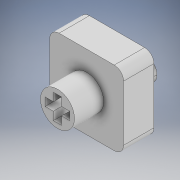
# Autodesk Inventor part: IPC CRUS 5 key
Saved by Autodesk Inventor 2022 (Build 260153000, 153)
## iProperties
Created: 2021-12-31
Part Number: IPC CRUS 5 key
Material: Generic
Document SubType Name: Modeling
Designer: solor
Density: 1 g/cm^3
Appearance: Default
Author: solor
Autodesk Inventor part; units mm, degrees
ref_plane "YZ Plane" through (0, 0, 0) normal (1, 0, 0) x (0, 1, 0)
ref_plane "XZ Plane" through (0, 0, 0) normal (0, 1, 0) x (-1, 0, 0)
sketch "Sketch1" plane through (0, 0, 0) normal (0, 0, 1) x (1, 0, 0)
  line L0 (14.6962, 12.74) -> (14.6962, 0) construction
  line L1 (10.61, 12.2) -> (1.53, 12.2)
  arc A0 (1.53, 12.2) -> (0, 10.67) centre (1.53, 10.67) ccw
  line L2 (0, 10.67) -> (0, 1.53)
  arc A1 (0, 1.53) -> (1.53, 0) centre (1.53, 1.53) ccw
  line L3 (1.53, 0) -> (10.61, 0)
  arc A2 (10.61, 0) -> (12.14, 1.53) centre (10.61, 1.53) ccw
  arc A3 (12.14, 10.67) -> (10.61, 12.2) centre (10.61, 10.67) ccw
  line L4 (12.14, 10.67) -> (12.14, 1.53)
  point P0 (0, 0)
  point P1 (0, 0)
  dimension "d10" = 12.74
  constraints: 10 end point, 8 point on circle, 4 centre point, 2 vertical, 1 point on line
  measures "d10" distance of L0.start L0.end
ref_plane "Work Plane1" through (0, 0, 5) normal (0, 0, 1) x (1, 0, 0)
sketch "Sketch2" plane through (0, 0, 5) normal (0, 0, 1) x (1, 0, 0)
  line L0 (10.88, 12.74) -> (1.8, 12.74) projected
  line L1 (10.88, 12.74) -> (1.8, 12.74) projected
  arc A0 (1.8, 12.74) -> (0, 10.94) centre (1.8, 10.94) ccw projected
  line L2 (0, 10.94) -> (0, 1.8) projected
  arc A1 (0, 1.8) -> (1.8, 0) centre (1.8, 1.8) ccw projected
  line L3 (1.8, 0) -> (10.88, 0) projected
  arc A2 (10.88, 0) -> (12.68, 1.8) centre (10.88, 1.8) ccw projected
  line L4 (12.68, 1.8) -> (12.68, 10.94) projected
  arc A3 (12.68, 10.94) -> (10.88, 12.74) centre (10.88, 10.94) ccw projected
  circle A4 centre (6.34, 6.37) radius 2.8
  line L5 (5.665, 8.395) -> (7.015, 8.395)
  line L6 (7.015, 4.345) -> (5.665, 4.345)
  line L7 (5.665, 4.345) -> (7.015, 8.395) construction
  line L8 (5.665, 8.395) -> (7.015, 4.345) construction
  line L9 (8.365, 5.695) -> (8.365, 7.045)
  line L10 (4.315, 7.045) -> (4.315, 5.695)
  line L11 (4.315, 5.695) -> (8.365, 7.045) construction
  line L12 (8.365, 5.695) -> (4.315, 7.045) construction
  line L13 (4.315, 5.695) -> (5.665, 5.695)
  line L14 (7.015, 5.695) -> (8.365, 5.695)
  line L15 (5.665, 4.345) -> (5.665, 5.695)
  line L16 (5.665, 7.045) -> (5.665, 8.395)
  line L17 (8.365, 7.045) -> (7.015, 7.045)
  line L18 (5.665, 7.045) -> (4.315, 7.045)
  line L19 (7.015, 8.395) -> (7.015, 7.045)
  line L20 (7.015, 5.695) -> (7.015, 4.345)
  point P0 (0, 0)
  dimension "d3" = 5.6
  dimension "d4" = 4.05
  dimension "d5" = 1.35
  dimension "d6" = 4.05
  dimension "d7" = 1.35
  constraints: 32 end point, 10 parallel, 8 perpendicular, 4 midpoint, 2 vertical, 1 centre point
  measures "d3" diameter of A4
  measures "d4" distance of L6.end L5.start
  measures "d5" distance of L5.start L5.end
  measures "d6" distance of L10.end L9.start
  measures "d7" distance of L9.end L9.start
extrude "Extrusion3" add sketch "Sketch1" along normal blind 5
sketch "Sketch3" plane through (0, 0, 5) normal (0, 0, 1) x (1, 0, 0)
  line L0 (10.61, 12.47) -> (1.53, 12.47)
  line L1 (10.61, 12.47) -> (1.53, 12.47)
  arc A0 (1.53, 12.47) -> (-0.27, 10.67) centre (1.53, 10.67) ccw
  line L2 (-0.27, 10.67) -> (-0.27, 1.53)
  arc A1 (-0.27, 1.53) -> (1.53, -0.27) centre (1.53, 1.53) ccw
  line L3 (1.53, -0.27) -> (10.61, -0.27)
  arc A2 (10.61, -0.27) -> (12.41, 1.53) centre (10.61, 1.53) ccw
  line L4 (12.41, 1.53) -> (12.41, 10.67)
  arc A3 (12.41, 10.67) -> (10.61, 12.47) centre (10.61, 10.67) ccw
  circle A4 centre (6.07, 6.1) radius 2.8
  line L5 (5.395, 8.125) -> (6.745, 8.125)
  line L6 (6.745, 4.075) -> (5.395, 4.075)
  line L7 (5.395, 4.075) -> (6.745, 8.125) construction
  line L8 (5.395, 8.125) -> (6.745, 4.075) construction
  line L9 (8.095, 5.425) -> (8.095, 6.775)
  line L10 (4.045, 6.775) -> (4.045, 5.425)
  line L11 (4.045, 5.425) -> (8.095, 6.775) construction
  line L12 (8.095, 5.425) -> (4.045, 6.775) construction
  line L13 (4.045, 5.425) -> (5.395, 5.425)
  line L14 (6.745, 5.425) -> (8.095, 5.425)
  line L15 (5.395, 4.075) -> (5.395, 5.425)
  line L16 (5.395, 6.775) -> (5.395, 8.125)
  line L17 (8.095, 6.775) -> (6.745, 6.775)
  line L18 (5.395, 6.775) -> (4.045, 6.775)
  line L19 (6.745, 8.125) -> (6.745, 6.775)
  line L20 (6.745, 5.425) -> (6.745, 4.075)
  line L21 (10.61, 12.2) -> (1.53, 12.2) projected
  line L22 (0, 10.67) -> (0, 1.53) projected
  point P0 (0, 0)
  point P1 (-0.27, -0.27)
  point P2 (6.07, 12.2)
  point P3 (0, 6.1)
  point P4 (6.07, 6.1)
  dimension "d14" = 5.6
  dimension "d15" = 4.05
  dimension "d16" = 1.35
  dimension "d17" = 4.05
  dimension "d18" = 1.35
  constraints: 42 end point, 10 parallel, 8 perpendicular, 8 point on circle, 6 midpoint, 5 centre point, 2 vertical
  measures "d14" diameter of A4
  measures "d15" distance of L6.end L5.start
  measures "d16" distance of L5.start L5.end
  measures "d17" distance of L10.end L9.start
  measures "d18" distance of L9.end L9.start
extrude "Extrusion4" add sketch "Sketch3" along normal blind 4.8 contours A4
sketch "Sketch4" plane through (0, 0, 0) normal (0, 0, -1) x (-1, 0, 0)
  line L0 (-13.9436, 0) -> (-13.9436, 2.266)
  line L1 (-15.5559, 0) -> (-15.5559, 6.84)
  line L2 (-1.53, 0) -> (-10.61, 0) projected
  line L3 (-11.8709, 10.0136) -> (-0.2691, 10.0136) construction
  line L4 (-0.2691, 10.0136) -> (-0.2691, 6.84) construction
  line L5 (-0.2691, 6.84) -> (-11.8709, 6.84) construction
  line L6 (-11.8709, 6.84) -> (-11.8709, 10.0136) construction
  line L7 (-7.4059, 5.3803) -> (-4.7341, 5.3803) construction
  line L8 (-4.7341, 5.3803) -> (-4.7341, 2.266) construction
  line L9 (-4.7341, 2.266) -> (-7.4059, 2.266) construction
  line L10 (-7.4059, 2.266) -> (-7.4059, 5.3803) construction
  spline S0 degree 2 poles (-10.2397, 6.8449) (-10.9268, 6.8449) (-11.7325, 7.6754) (-11.7325, 8.4268) knots 0 0 0 1 2 2 2
  spline S1 degree 2 poles (-11.7325, 8.4268) (-11.7325, 9.151) (-10.9243, 10.0136) (-10.2372, 10.0136) knots 0 0 0 1 2 2 2
  spline S2 degree 2 poles (-10.2372, 10.0136) (-10.0568, 10.0136) (-9.7651, 9.9716) (-9.6316, 9.937) knots 0 0 0 1 2 2 2
  spline S3 degree 2 poles (-9.6316, 9.937) (-9.5278, 9.9048) (-9.2831, 9.7985) (-9.2065, 9.759) knots 0 0 0 1 2 2 2
  line L11 (-9.2065, 9.759) -> (-9.2065, 9.0323)
  line L12 (-9.2065, 9.0323) -> (-9.2831, 9.0323)
  spline S4 degree 2 poles (-9.2831, 9.0323) (-9.34, 9.0818) (-9.508, 9.2202) (-9.6143, 9.2844) knots 0 0 0 1 2 2 2
  spline S5 degree 2 poles (-9.6143, 9.2844) (-9.7206, 9.3512) (-9.9752, 9.4426) (-10.1161, 9.4426) knots 0 0 0 1 2 2 2
  spline S6 degree 2 poles (-10.1161, 9.4426) (-10.2817, 9.4426) (-10.556, 9.3388) (-10.6821, 9.2078) knots 0 0 0 1 2 2 2
  spline S7 degree 2 poles (-10.6821, 9.2078) (-10.7958, 9.0917) (-10.9416, 8.6937) (-10.9416, 8.4243) knots 0 0 0 1 2 2 2
  spline S8 degree 2 poles (-10.9416, 8.4243) (-10.9416, 8.1401) (-10.7908, 7.752) (-10.6672, 7.6334) knots 0 0 0 1 2 2 2
  spline S9 degree 2 poles (-10.6672, 7.6334) (-10.5486, 7.5172) (-10.257, 7.4159) (-10.1111, 7.4159) knots 0 0 0 1 2 2 2
  spline S10 degree 2 poles (-10.1111, 7.4159) (-9.9604, 7.4159) (-9.686, 7.5172) (-9.5921, 7.579) knots 0 0 0 1 2 2 2
  spline S11 degree 2 poles (-9.5921, 7.579) (-9.4883, 7.6408) (-9.3326, 7.7718) (-9.2757, 7.8237) knots 0 0 0 1 2 2 2
  line L13 (-9.2757, 7.8237) -> (-9.2065, 7.8237)
  line L14 (-9.2065, 7.8237) -> (-9.2065, 7.1069)
  spline S12 degree 2 poles (-9.2065, 7.1069) (-9.2905, 7.0674) (-9.5105, 6.9685) (-9.6292, 6.9339) knots 0 0 0 1 2 2 2
  spline S13 degree 2 poles (-9.6292, 6.9339) (-9.7725, 6.8894) (-10.0221, 6.8449) (-10.2397, 6.8449) knots 0 0 0 1 2 2 2
  line L15 (-5.9365, 6.9043) -> (-6.8683, 6.9043)
  line L16 (-6.8683, 6.9043) -> (-7.7161, 8.0239)
  line L17 (-7.7161, 8.0239) -> (-7.9929, 8.0239)
  line L18 (-7.9929, 8.0239) -> (-7.9929, 6.9043)
  line L19 (-7.9929, 6.9043) -> (-8.7542, 6.9043)
  line L20 (-8.7542, 6.9043) -> (-8.7542, 9.9543)
  line L21 (-8.7542, 9.9543) -> (-7.5283, 9.9543)
  spline S14 degree 2 poles (-7.5283, 9.9543) (-7.2737, 9.9543) (-6.898, 9.89) (-6.7373, 9.7911) knots 0 0 0 1 2 2 2
  spline S15 degree 2 poles (-6.7373, 9.7911) (-6.5742, 9.6873) (-6.3814, 9.3635) (-6.3814, 9.1164) knots 0 0 0 1 2 2 2
  spline S16 degree 2 poles (-6.3814, 9.1164) (-6.3814, 8.7679) (-6.6978, 8.3304) (-6.9623, 8.2019) knots 0 0 0 1 2 2 2
  line L22 (-6.9623, 8.2019) -> (-5.9365, 6.9043)
  spline S17 degree 2 poles (-7.1674, 9.02) (-7.1674, 9.1362) (-7.2564, 9.3018) (-7.3577, 9.3462) knots 0 0 0 1 2 2 2
  spline S18 degree 2 poles (-7.3577, 9.3462) (-7.4294, 9.3759) (-7.6049, 9.3932) (-7.7359, 9.3932) knots 0 0 0 1 2 2 2
  line L23 (-7.7359, 9.3932) -> (-7.9929, 9.3932)
  line L24 (-7.9929, 9.3932) -> (-7.9929, 8.5726)
  line L25 (-7.9929, 8.5726) -> (-7.773, 8.5726)
  spline S19 degree 2 poles (-7.773, 8.5726) (-7.6148, 8.5726) (-7.3899, 8.6122) (-7.3132, 8.674) knots 0 0 0 1 2 2 2
  spline S20 degree 2 poles (-7.3132, 8.674) (-7.2391, 8.7333) (-7.1674, 8.8915) (-7.1674, 9.02) knots 0 0 0 1 2 2 2
  spline S21 degree 2 poles (-4.4758, 6.84) (-5.0912, 6.84) (-5.7536, 7.4332) (-5.7536, 8.0066) knots 0 0 0 1 2 2 2
  line L26 (-5.7536, 8.0066) -> (-5.7536, 9.9543)
  line L27 (-5.7536, 9.9543) -> (-4.9874, 9.9543)
  line L28 (-4.9874, 9.9543) -> (-4.9874, 8.0511)
  spline S22 degree 2 poles (-4.9874, 8.0511) (-4.9874, 7.7323) (-4.7477, 7.4208) (-4.4758, 7.4208) knots 0 0 0 1 2 2 2
  spline S23 degree 2 poles (-4.4758, 7.4208) (-4.2113, 7.4208) (-3.9642, 7.7199) (-3.9642, 8.0511) knots 0 0 0 1 2 2 2
  line L29 (-3.9642, 8.0511) -> (-3.9642, 9.9543)
  line L30 (-3.9642, 9.9543) -> (-3.198, 9.9543)
  line L31 (-3.198, 9.9543) -> (-3.198, 8.0091)
  spline S24 degree 2 poles (-3.198, 8.0091) (-3.198, 7.4456) (-3.8431, 6.84) (-4.4758, 6.84) knots 0 0 0 1 2 2 2
  spline S25 degree 2 poles (-1.668, 6.8499) (-2.019, 6.8499) (-2.5479, 6.9858) (-2.7753, 7.0847) knots 0 0 0 1 2 2 2
  line L32 (-2.7753, 7.0847) -> (-2.7753, 7.8114)
  line L33 (-2.7753, 7.8114) -> (-2.7061, 7.8114)
  spline S26 degree 2 poles (-2.7061, 7.8114) (-2.4762, 7.6161) (-1.9251, 7.406) (-1.6655, 7.406) knots 0 0 0 1 2 2 2
  spline S27 degree 2 poles (-1.6655, 7.406) (-1.5988, 7.406) (-1.3838, 7.4357) (-1.3195, 7.4653) knots 0 0 0 1 2 2 2
  spline S28 degree 2 poles (-1.3195, 7.4653) (-1.2404, 7.4999) (-1.1292, 7.626) (-1.1292, 7.7273) knots 0 0 0 1 2 2 2
  spline S29 degree 2 poles (-1.1292, 7.7273) (-1.1292, 7.8435) (-1.3096, 7.9868) (-1.4332, 8.019) knots 0 0 0 1 2 2 2
  spline S30 degree 2 poles (-1.4332, 8.019) (-1.5889, 8.061) (-1.9424, 8.1327) (-2.0981, 8.187) knots 0 0 0 1 2 2 2
  spline S31 degree 2 poles (-2.0981, 8.187) (-2.4515, 8.3106) (-2.758, 8.7333) (-2.758, 9.0496) knots 0 0 0 1 2 2 2
  spline S32 degree 2 poles (-2.758, 9.0496) (-2.758, 9.4772) (-2.0338, 10.0086) (-1.4901, 10.0086) knots 0 0 0 1 2 2 2
  spline S33 degree 2 poles (-1.4901, 10.0086) (-1.2182, 10.0086) (-0.6794, 9.8974) (-0.4668, 9.8035) knots 0 0 0 1 2 2 2
  line L34 (-0.4668, 9.8035) -> (-0.4668, 9.1065)
  line L35 (-0.4668, 9.1065) -> (-0.5335, 9.1065)
  spline S34 degree 2 poles (-0.5335, 9.1065) (-0.7041, 9.2523) (-1.1935, 9.4525) (-1.4505, 9.4525) knots 0 0 0 1 2 2 2
  spline S35 degree 2 poles (-1.4505, 9.4525) (-1.5518, 9.4525) (-1.71, 9.4229) (-1.799, 9.3833) knots 0 0 0 1 2 2 2
  spline S36 degree 2 poles (-1.799, 9.3833) (-1.8707, 9.3512) (-1.9745, 9.2227) (-1.9745, 9.1436) knots 0 0 0 1 2 2 2
  spline S37 degree 2 poles (-1.9745, 9.1436) (-1.9745, 9.0249) (-1.8089, 8.889) (-1.5716, 8.8346) knots 0 0 0 1 2 2 2
  spline S38 degree 2 poles (-1.5716, 8.8346) (-1.4184, 8.8) (-1.1341, 8.7333) (-0.971, 8.6764) knots 0 0 0 1 2 2 2
  spline S39 degree 2 poles (-0.971, 8.6764) (-0.6546, 8.5603) (-0.3457, 8.1747) (-0.3457, 7.8583) knots 0 0 0 1 2 2 2
  spline S40 degree 2 poles (-0.3457, 7.8583) (-0.3457, 7.4035) (-1.06, 6.8499) (-1.668, 6.8499) knots 0 0 0 1 2 2 2
  spline S41 degree 2 poles (-4.9244, 3.3634) (-4.9244, 3.1237) (-5.0875, 2.7183) (-5.2482, 2.5725) knots 0 0 0 1 2 2 2
  spline S42 degree 2 poles (-5.2482, 2.5725) (-5.4088, 2.4267) (-5.8488, 2.266) (-6.1701, 2.266) knots 0 0 0 1 2 2 2
  spline S43 degree 2 poles (-6.1701, 2.266) (-6.5112, 2.2685) (-7.0006, 2.3797) (-7.1612, 2.4514) knots 0 0 0 1 2 2 2
  line L36 (-7.1612, 2.4514) -> (-7.1612, 3.1162)
  line L37 (-7.1612, 3.1162) -> (-7.092, 3.1162)
  spline S44 degree 2 poles (-7.092, 3.1162) (-7.0327, 3.0841) (-6.8893, 3.0001) (-6.7732, 2.9556) knots 0 0 0 1 2 2 2
  spline S45 degree 2 poles (-6.7732, 2.9556) (-6.6644, 2.9136) (-6.4395, 2.8567) (-6.3036, 2.8567) knots 0 0 0 1 2 2 2
  spline S46 degree 2 poles (-6.3036, 2.8567) (-6.1849, 2.8567) (-5.9081, 2.916) (-5.8241, 2.9951) knots 0 0 0 1 2 2 2
  spline S47 degree 2 poles (-5.8241, 2.9951) (-5.7623, 3.0569) (-5.6931, 3.2077) (-5.6931, 3.3337) knots 0 0 0 1 2 2 2
  spline S48 degree 2 poles (-5.6931, 3.3337) (-5.6931, 3.4425) (-5.7821, 3.5957) (-5.8537, 3.6427) knots 0 0 0 1 2 2 2
  spline S49 degree 2 poles (-5.8537, 3.6427) (-5.9575, 3.7119) (-6.2541, 3.7515) (-6.3604, 3.7515) knots 0 0 0 1 2 2 2
  spline S50 degree 2 poles (-6.3604, 3.7515) (-6.5285, 3.7515) (-6.8473, 3.6971) (-6.9635, 3.6674) knots 0 0 0 1 2 2 2
  line L38 (-6.9635, 3.6674) -> (-7.0302, 3.6674)
  line L39 (-7.0302, 3.6674) -> (-7.0302, 5.3803)
  line L40 (-7.0302, 5.3803) -> (-5.0084, 5.3803)
  line L41 (-5.0084, 5.3803) -> (-5.0084, 4.8044)
  line L42 (-5.0084, 4.8044) -> (-6.306, 4.8044)
  line L43 (-6.306, 4.8044) -> (-6.306, 4.2977)
  spline S51 degree 2 poles (-6.306, 4.2977) (-6.2443, 4.3026) (-6.0737, 4.3076) (-6.0267, 4.3076) knots 0 0 0 1 2 2 2
  spline S52 degree 2 poles (-6.0267, 4.3076) (-5.8068, 4.3076) (-5.436, 4.2186) (-5.2902, 4.1271) knots 0 0 0 1 2 2 2
  spline S53 degree 2 poles (-5.2902, 4.1271) (-5.1172, 4.0134) (-4.9244, 3.6353) (-4.9244, 3.3634) knots 0 0 0 1 2 2 2
  point P0 (0, 0)
  point P1 (-6.07, 0)
  point P2 (-6.07, 2.266)
  point P3 (-6.07, 6.84)
  point P4 (-6.07, 6.84)
  point P5 (-6.07, 2.266)
  dimension "d21" = 2.266
  dimension "d22" = 6.84
  constraints: 4 end point, 3 midpoint, 2 vertical, 4 other
  measures "d21" distance of L0.start L0.end
  measures "d22" distance of L1.start L1.end
extrude "Extrusion5" add sketch "Sketch4" along normal blind 0.9
body "Solid2"
